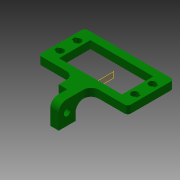
# Autodesk Inventor part: TopBar
Saved by Autodesk Inventor 2014 SP1 (Build 180222100, 222)
## iProperties
Created: 2017-01-18
Part Number: TopBar
Material: Generic
Document SubType Name: Modeling
Designer: danielsikar
Density: 1 g/cm^3
Appearance: Dark Green
Author: danielsikar
Autodesk Inventor part; units mm, degrees
ref_plane "YZ Plane" through (0, 0, 0) normal (1, 0, 0) x (0, 1, 0)
ref_plane "XZ Plane" through (0, 0, 0) normal (0, 1, 0) x (-1, 0, 0)
sketch "Sketch1" plane through (0, 0, 0) normal (0, 0, 1) x (1, 0, 0)
  line L0 (0, 0) -> (-6.8, 0)
  line L1 (-6.8, 0) -> (-6.8, 20)
  line L2 (-6.8, 20) -> (0, 20)
  line L3 (0, 20) -> (0, 0)
  line L4 (-5.8439, 5.5) -> (-6.8, 5.5) projected
  line L5 (-6.8, 14.5) -> (-6.8, 5.5) projected
  line L6 (-6.8, 14.5) -> (-5.8439, 14.5) projected
  arc A0 (-5.8439, 14.5) -> (-5.8439, 16.9) centre (-4, 15.7) ccw projected
  line L7 (-5.8439, 16.9) -> (-6.8, 16.9) projected
  line L8 (-6.8, 20) -> (-6.8, 16.9) projected
  line L9 (0, 20) -> (-6.8, 20) projected
  line L10 (0, 0) -> (0, 20) projected
  line L11 (0, 0) -> (-6.8, 0) projected
  line L12 (-6.8, 3.1) -> (-6.8, 0) projected
  line L13 (-6.8, 3.1) -> (-5.8439, 3.1) projected
  arc A1 (-5.8439, 3.1) -> (-5.8439, 5.5) centre (-4, 4.3) ccw projected
  dimension "d0" = 6.8
  dimension "d1" = 20
  constraints: 8 end point, 2 parallel, 1 horizontal, 1 perpendicular
  measures "d0" distance of L1.end L2.end
  measures "d1" distance of L0.end L1.end
extrude "Extrusion1" add sketch "Sketch1" along normal blind 5 contours L0 L1 L13 A1 L4 L6 A0 L7 L2 L3
ref_plane "Work Plane1" through (20.15, 10, -1.65) normal (-1, 0, 0) x (0, 1, 0)
mirror "Mirror1" about plane through (20.15, 10, -1.65) normal (-1, 0, 0) of "Extrusion1"
sketch "Sketch2" plane through (-6.8, 0, 0) normal (0, -1, 0) x (1, 0, 0)
  line L0 (0, 0) -> (53.9, 0)
  line L1 (53.9, 0) -> (53.9, 5)
  line L2 (53.9, 5) -> (0, 5)
  line L3 (0, 5) -> (0, 0)
  dimension "d4" = 53.9
  constraints: 8 end point, 2 parallel, 1 horizontal, 1 perpendicular
  measures "d4" distance of L2.end L1.end
extrude "Extrusion2" add sketch "Sketch2" along normal blind 5
sketch "Sketch3" plane through (-6.8, 3.1, 0) normal (-1, 0, 0) x (0, 0, 1)
  line L0 (0, -8.1) -> (5, -8.1)
  line L1 (5, -8.1) -> (5, 16.9)
  line L2 (5, 16.9) -> (0, 16.9)
  line L3 (0, 16.9) -> (0, -8.1)
  point P0 (0, -3.1)
  dimension "d7" = 25
  constraints: 8 end point, 2 parallel, 1 horizontal, 1 perpendicular
  measures "d7" distance of L1.end L0.end
extrude "Extrusion3" add sketch "Sketch3" along normal blind 2
mirror "Mirror2" about plane through (20.15, 10, -1.65) normal (-1, 0, 0) of "Extrusion3"
fillet "Fillet1" radius 2 1 edges at (-8.8, -5, 2.5)
fillet "Fillet2" radius 2 1 edges at (49.1, -5, 2.5)
sketch "Sketch4" plane through (0, 20, 5) normal (1, 0, 0) x (0, 0, -1)
  line L0 (5, -20) -> (5, 0) projected
  line L1 (5, 0) -> (0, 0) projected
  line L2 (0, -20) -> (0, 0) projected
  line L3 (5, -20) -> (0, -20) projected
extrude "Extrusion4" cut sketch "Sketch4" against normal blind 0.25
mirror "Mirror3" about plane through (20.15, 10, -1.65) normal (-1, 0, 0) of "Extrusion4"
sketch "Sketch5" plane through (-8.8, 20, 5) normal (0, 1, 0) x (1, 0, 0)
  line L0 (0, 0) -> (57.9, 0)
  line L1 (57.9, 0) -> (57.9, 5)
  line L2 (57.9, 5) -> (0, 5)
  line L3 (0, 5) -> (0, 0)
  point P0 (8.8, 5)
  dimension "d14" = 57.9
  constraints: 8 end point, 2 parallel, 1 horizontal, 1 perpendicular
  measures "d14" distance of L2.end L1.end
extrude "Extrusion5" add sketch "Sketch5" along normal blind 5
sketch "Sketch6" plane through (-8.8, 20, 5) normal (0, -1, 0) x (1, 0, 0)
  line L0 (8.55, 0) -> (8.55, -5) projected
  line L1 (49.35, -5) -> (8.55, -5) projected
  line L2 (49.35, -5) -> (49.35, 0) projected
  line L3 (8.55, 0) -> (49.35, 0) projected
  point P0 (8.8, -5)
extrude "Extrusion6" cut sketch "Sketch6" against normal blind 0.15
sketch "Sketch7" plane through (-6.8, 0, 0) normal (0, 1, 0) x (1, 0, 0)
  line L0 (47.35, -5) -> (6.55, -5) projected
  line L1 (47.35, 0) -> (47.35, -5) projected
  line L2 (6.55, 0) -> (47.35, 0) projected
  line L3 (6.55, 0) -> (6.55, -5) projected
  point P0 (6.8, 0)
extrude "Extrusion7" cut sketch "Sketch7" against normal blind 0.15
sketch "Sketch9" plane through (-6.8, -5, 0) normal (0, -1, 0) x (1, 0, 0)
  line L0 (0, 5) -> (53.9, 5) projected
  line L1 (53.9, 0) -> (0, 0) projected
  line L2 (26.65, -10.0707) -> (26.65, 15.0707) construction
  line L3 (55.9, 0) -> (55.9, 5) construction
  line L4 (21.15, 5) -> (32.15, 5)
  line L5 (32.15, 5) -> (32.15, 0)
  line L6 (32.15, 0) -> (21.15, 0)
  line L7 (21.15, 0) -> (21.15, 5)
  point P0 (6.8, 0)
  dimension "d23" = 29.25
  dimension "d24" = 11
  dimension "d25" = 5.5
  constraints: 10 end point, 2 parallel, 2 perpendicular, 2 point on line, 1 horizontal
  measures "d23" distance between parallel lines of L2 L3
  measures "d24" distance of L5.end L6.end
  measures "d25" distance between parallel lines of L5 L2
extrude "Extrusion9" add sketch "Sketch9" along normal blind 21
fillet "Fillet3" radius 5 2 edges at (14.35, -5, 2.5) (25.35, -5, 2.5)
sketch "Sketch10" plane through (0, 0, 0) normal (0, 0, -1) x (-1, 0, 0)
  line L0 (-47.1, -5) -> (-30.35, -5) projected
  line L1 (-14.35, -10) -> (-14.35, -26) projected
  line L2 (-25.35, -15) -> (-19.85, -15)
  line L3 (-19.85, -15) -> (-19.85, -26)
  line L4 (-19.85, -26) -> (-25.35, -26)
  line L5 (-25.35, -10) -> (-25.35, -26) projected
  line L6 (-9.35, -5) -> (6.8, -5) projected
  line L7 (-25.35, -15) -> (-25.35, -26)
  point P0 (0, 0)
  dimension "d30" = 11
  dimension "d31" = 10
  dimension "d32" = 5.5
  constraints: 8 end point, 2 perpendicular, 2 point on line, 1 horizontal, 1 parallel
  measures "d30" distance of L2.end L3.end
  measures "d31" distance between parallel lines of L2 L0
  measures "d32" distance between parallel lines of L1 L3
extrude "Extrusion10" add sketch "Sketch10" along normal blind 10
fillet "Fillet7" radius 5 1 edges at (22.6, -15, 0)
sketch "Sketch11" plane through (0, 0, 0) normal (0, 0, -1) x (-1, 0, 0)
  line L0 (-19.85, -10) -> (-19.85, -26) projected
  line L1 (-14.35, -26) -> (-19.85, -26)
  line L2 (-19.85, -26) -> (-19.85, -15)
  line L3 (-19.85, -15) -> (-14.35, -15)
  line L4 (-14.35, -15) -> (-14.35, -26)
  point P0 (0, 0)
  dimension "d39" = 11
  constraints: 8 end point, 2 parallel, 1 horizontal, 1 perpendicular, 1 point on line
  measures "d39" distance of L1.end L2.end
extrude "Extrusion11" cut sketch "Sketch11" against normal blind 10
sketch "Sketch12" plane through (25.35, -26, 5) normal (1, 0, 0) x (0, 0, -1)
  line L0 (15, 11) -> (15, 0) projected
  circle A0 centre (7.5, 5.5) radius 2.15
  point P0 (5, 26)
  dimension "d42" = 4.3
  dimension "d43" = 7.5
  constraints: 1 centre point
  measures "d42" diameter of A0
  measures "d43" distance from line of A0.centre L0
extrude "Extrusion12" cut sketch "Sketch12" against normal blind 10
fillet "Fillet8" radius 5 1 edges at (22.6, -26, 5)
sketch "Sketch14" plane through (20.15, 10, -1.65) normal (1, 0, 0) x (0, 1, 0)
  point P0 (-10, -1.65)
fillet "Fillet9" radius 2 2 edges at (49.1, 25, 2.5) (-8.8, 25, 2.5)
ref_plane "Work Plane2" through (20.15, 10, -1.65) normal (-1, 0, 0) x (0, 1, 0)
body "Solid1"
